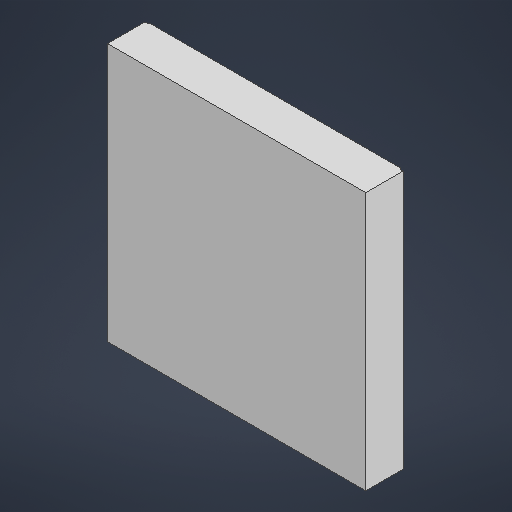
# Autodesk Inventor part: 零件1
Saved by Autodesk Inventor 2025 (Build 290162000, 162)
## iProperties
Created: 2025-06-18
Part Number: 零件1
Material: 常规
Document SubType Name: Modeling
Designer: XH
Density: 1 g/cm^3
Appearance: 默认
Author: XH
Autodesk Inventor part; units mm, degrees
ref_plane "YZ Plane" through (0, 0, 0) normal (1, 0, 0) x (0, 1, 0)
ref_plane "XZ Plane" through (0, 0, 0) normal (0, 1, 0) x (-1, 0, 0)
ref_plane "XY Plane" through (0, 0, 0) normal (0, 0, 1) x (1, 0, 0)
sketch "草图1" plane through (0, 0, 0) normal (0, 0, 1) x (1, 0, 0)
  line L0 (485, -500) -> (-485, -500)
  line L1 (-485, -500) -> (-485, 500)
  line L2 (-485, 500) -> (485, 500)
  line L3 (485, 500) -> (485, -500)
  line L4 (485, -500) -> (-485, 500) construction
  line L5 (-485, -500) -> (485, 500) construction
  point P0 (0, 0)
  dimension "d0" = 1000
  dimension "d1" = 970
  constraints: 12 end point, 2 midpoint, 2 parallel, 1 horizontal, 1 perpendicular
  measures "d0" distance of L0.end L1.end
  measures "d1" distance of L1.end L2.end
extrude "拉伸1" add sketch "草图1" along normal blind 5
sketch "草图2" plane through (0, 0, 5) normal (0, 0, 1) x (1, 0, 0)
  line L0 (500, -500) -> (-500, -500)
  line L1 (-500, -500) -> (-500, 500)
  line L2 (-500, 500) -> (500, 500)
  line L3 (500, 500) -> (500, -500)
  line L4 (500, -500) -> (-500, 500) construction
  line L5 (-500, -500) -> (500, 500) construction
  line L6 (485, 500) -> (-485, 500) projected
  line L7 (-485, 500) -> (-485, -500) projected
  point P0 (0, 0)
  point P1 (-485, 500)
  dimension "d5" = 1000
  constraints: 12 end point, 2 midpoint, 2 parallel, 1 collinear, 1 horizontal, 1 perpendicular
  measures "d5" distance between parallel lines of L3 L1
extrude "拉伸2" add sketch "草图2" along normal blind 145
chamfer "倒角1" distance 4 distance2 5 1 edges at (-485, 0, 5) measured on face at (-485.5, 0, 5)
chamfer "倒角2" distance 4 distance2 5 1 edges at (485, 0, 5) measured on face at (485.5, 0, 5)
